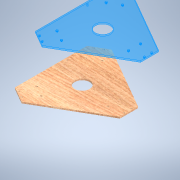
# Autodesk Inventor part: lep_felso
Saved by Autodesk Inventor 2022 (Build 260153000, 153)
## iProperties
Created: 2021-10-06
Part Number: lep_felso
Material: Wood (Birch)
Document SubType Name: Modeling
Designer: Varga Tamás
Density: 0.55 g/cm^3
Appearance: Birch - Natural Polished
Mass: 135.42 g
Surface Area: 1049.92 cm^2
Volume: 246.217 cm^3
Author: Varga Tamás
Autodesk Inventor part; units mm, degrees
ref_plane "YZ Plane" through (0, 0, 0) normal (1, 0, 0) x (0, 1, 0)
ref_plane "XZ Plane" through (0, 0, 0) normal (0, 1, 0) x (-1, 0, 0)
ref_plane "XY Plane" through (0, 0, 0) normal (0, 0, 1) x (1, 0, 0)
sketch "Sketch1" plane through (0, 0, 0) normal (0, 1, 0) x (-1, 0, 0)
  line L0 (-259.8076, 150) -> (-259.8076, 90)
  line L1 (-259.8076, 90) -> (-51.9615, -30)
  line L2 (-51.9615, -30) -> (0, 0)
  line L3 (0, 0) -> (0, 240)
  line L4 (0, 240) -> (-51.9615, 270)
  line L5 (-51.9615, 270) -> (-259.8076, 150)
  dimension "d0" = 120
  dimension "d1" = 120
  dimension "d2" = 120
  dimension "d4" = 120
  dimension "d5" = 120
  dimension "d6" = 60
  dimension "d7" = 120
  constraints: 13 end point, 2 equal length, 1 vertical
  measures "d0" angle of L4 L5
  measures "d1" angle of L3 L2
  measures "d2" angle of L1 L0
  measures "d4" angle of L1 L2
  measures "d5" angle of L3 L4
  measures "d6" distance of L0.start L0.end
  measures "d7" vertical distance of L4.end L0.start
extrude "Extrusion1" add sketch "Sketch1" along normal blind 5
sketch "Sketch2" plane through (0, 5, 0) normal (0, 1, 0) x (1, 0, 0)
  line L0 (254.8076, -108) -> (254.8076, -132)
  line L1 (259.8076, -150) -> (259.8076, -90) projected
  line L2 (259.8076, -90) -> (51.9615, 30) projected
  line L3 (51.9615, -270) -> (259.8076, -150) projected
  line L4 (209.8076, -108) -> (209.8076, -132)
  line L5 (209.8076, -108) -> (209.8076, -100)
  line L6 (209.8076, -144.7569) -> (209.8076, -140)
  point P0 (0, 0)
  dimension "d10" = 24
  dimension "d11" = 5
  dimension "d12" = 18
  dimension "d31" = 18.0885
  dimension "d32" = 18.0885
  dimension "d33" = 18
  dimension "d44" = 45
  dimension "d45" = 0
  dimension "d47" = 40.5885
  dimension "d51" = 8
  dimension "d52" = 8
  constraints: 8 end point, 6 coincident, 3 vertical, 2 parallel, 1 collinear
  measures "d10" distance of L0.start L0.end
  measures "d11" distance between parallel lines of L1 L0
  measures "d12" vertical distance of L1.end L0.start
  measures "d31" distance from line of L2 L0.start
  measures "d32" distance from line of L3 L0.end
  measures "d33" vertical distance of L1.start L0.end
  measures "d44" distance between parallel lines of L0 L4
  measures "d45" vertical distance of L0.start L4.start
  measures "d47" distance from line of L2 L4.start
  measures "d51" distance of L5.start L5.end
  measures "d52" distance of point (209.808, -132) L6.end
hole "Hole1" at (209.8076, 5, 100) at (209.8076, 5, 140) at (254.8076, 5, 108) at (254.8076, 5, 132) direction (0, -1, 0) diameter 2.8 end through all
sketch "Sketch3" plane through (0, 5, 0) normal (0, 1, 0) x (1, 0, 0)
  line L0 (18.088, 4.6696) -> (38.8735, 16.6701)
  line L1 (51.9615, 30) -> (0, 0) projected
  line L2 (0, 0) -> (0, -240) projected
  line L3 (259.8076, -90) -> (51.9615, 30) projected
  line L4 (47.516, -30.3017) -> (68.3015, -18.3011)
  line L5 (68.3015, -18.3011) -> (68.3015, -18.3011)
  line L6 (47.516, -30.3017) -> (33.66, -38.3014)
  dimension "d20" = 5
  dimension "d22" = 18.088
  dimension "d23" = 18.088
  dimension "d46" = 45
  dimension "d48" = 33.66
  dimension "d53" = 33.66
  dimension "d89" = 33.66
  constraints: 8 end point, 6 coincident, 3 parallel, 2 collinear
  measures "d20" distance from line of L1.end L0
  measures "d22" distance from line of L0.start L2
  measures "d23" distance from line of L3 L0.end
  measures "d46" distance between parallel lines of L4 L0
  measures "d48" distance from line of L3 L4.end
  measures "d53" distance from line of L3 L5.end
  measures "d89" distance from line of L2 point (33.66, -38.301)
hole "Hole2" at (68.3015, 5, 18.3011) at (33.66, 5, 38.3014) at (18.088, 5, -4.6696) at (38.8735, 5, -16.6701) direction (0, -1, 0) diameter 2.8 end through all
sketch "Sketch4" plane through (0, 5, 0) normal (0, 1, 0) x (1, 0, 0)
  line L0 (18.088, -244.6696) -> (38.8735, -256.6701)
  line L1 (0, -240) -> (51.9615, -270) projected
  line L2 (51.9615, -270) -> (259.8076, -150) projected
  line L3 (0, 0) -> (0, -240) projected
  line L4 (47.516, -209.6983) -> (68.3015, -221.6989)
  line L5 (68.3015, -221.6989) -> (68.3015, -221.6989)
  line L6 (47.516, -209.6983) -> (33.66, -201.6986)
  dimension "d34" = 5
  dimension "d35" = 18.088
  dimension "d36" = 18.088
  dimension "d49" = 45
  dimension "d50" = 33.66
  dimension "d56" = 33.66
  dimension "d90" = 33.66
  constraints: 8 end point, 6 coincident, 3 parallel, 2 collinear
  measures "d34" distance between parallel lines of L1 L0
  measures "d35" distance from line of L2 L0.end
  measures "d36" distance from line of L3 L0.start
  measures "d49" distance between parallel lines of L4 L0
  measures "d50" distance from line of L2 L4.end
  measures "d56" distance from line of L2 L5.end
  measures "d90" distance from line of L3 point (33.66, -201.699)
hole "Hole3" at (68.3015, 5, 221.6989) at (33.66, 5, 201.6986) at (18.088, 5, 244.6696) at (38.8735, 5, 256.6701) direction (0, -1, 0) diameter 2.8 end through all
sketch "Sketch5" plane through (0, 5, 0) normal (0, 1, 0) x (1, 0, 0)
  circle A0 centre (103.923, -120) radius 25
  line L0 (0, 0) -> (0, -240) projected
  line L1 (259.8076, -90) -> (51.9615, 30) projected
  line L2 (51.9615, 30) -> (0, 0) projected
  line L3 (25.9808, 15) -> (155.8846, -210)
  line L4 (51.9615, -270) -> (259.8076, -150) projected
  line L5 (51.9615, 30) -> (0, 0) projected
  line L6 (0, 0) -> (0, -240) projected
  line L7 (0, -120) -> (259.8076, -120)
  line L8 (259.8076, -150) -> (259.8076, -90) projected
  line L9 (0, -240) -> (51.9615, -270) projected
  line L10 (25.9808, -255) -> (155.8846, -30)
  dimension "d57" = 50
  dimension "d60" = 0
  dimension "d61" = 0
  constraints: 6 end point, 6 midpoint, 2 perpendicular, 1 centre point
  measures "d57" diameter of A0
  measures "d60" distance from line of A0.centre L7
  measures "d61" distance from line of L3 A0.centre
extrude "Extrusion2" cut sketch "Sketch5" against normal through all contours L7 L10 A0 | A0 L3 L7 | L10 L3 A0 | A0 L10 L3 | L7 A0 L3 | L10 A0 L7
sketch "Sketch6" plane through (0, 5, 0) normal (0, 1, 0) x (1, 0, 0)
  circle A0 centre (103.923, -120) radius 25 projected
  circle A1 centre (18.088, -244.6696) radius 1.4 projected
  circle A2 centre (68.3015, -221.6989) radius 1.4 projected
  circle A3 centre (33.66, -201.6986) radius 1.4 projected
  circle A4 centre (38.8735, -256.6701) radius 1.4 projected
  circle A5 centre (18.088, 4.6696) radius 1.4 projected
  circle A6 centre (68.3015, -18.3011) radius 1.4 projected
  circle A7 centre (33.66, -38.3014) radius 1.4 projected
  circle A8 centre (38.8735, 16.6701) radius 1.4 projected
  circle A9 centre (254.8076, -108) radius 1.4 projected
  circle A10 centre (209.8076, -100) radius 1.4 projected
  circle A11 centre (209.8076, -140) radius 1.4 projected
  circle A12 centre (254.8076, -132) radius 1.4 projected
  line L0 (259.8076, -90) -> (51.9615, 30) projected
  line L1 (51.9615, 30) -> (0, 0) projected
  line L2 (0, 0) -> (0, -240) projected
  line L3 (0, -240) -> (51.9615, -270) projected
  line L4 (51.9615, -270) -> (259.8076, -150) projected
  line L5 (259.8076, -150) -> (259.8076, -90) projected
  line L6 (36.3641, -199.5334) -> (36.8871, -202.9578)
  line L7 (36.8871, -202.9578) -> (34.183, -205.123)
  line L8 (34.183, -205.123) -> (30.9559, -203.8638)
  line L9 (30.9559, -203.8638) -> (30.4329, -200.4394)
  line L10 (30.4329, -200.4394) -> (33.137, -198.2742)
  line L11 (33.137, -198.2742) -> (36.3641, -199.5334)
  circle A13 centre (68.3015, -221.6989) radius 1.4 projected
  line L12 (67.8588, -218.2632) -> (71.0556, -219.5976)
  line L13 (71.0556, -219.5976) -> (71.4983, -223.0333)
  line L14 (71.4983, -223.0333) -> (68.7442, -225.1346)
  line L15 (68.7442, -225.1346) -> (65.5475, -223.8001)
  line L16 (65.5475, -223.8001) -> (65.1048, -220.3644)
  line L17 (65.1048, -220.3644) -> (67.8588, -218.2632)
  circle A14 centre (209.8076, -140) radius 1.4 projected
  line L18 (212.8076, -138.2679) -> (212.8076, -141.7321)
  line L19 (212.8076, -141.7321) -> (209.8076, -143.4641)
  line L20 (209.8076, -143.4641) -> (206.8076, -141.7321)
  line L21 (206.8076, -141.7321) -> (206.8076, -138.2679)
  line L22 (206.8076, -138.2679) -> (209.8076, -136.5359)
  line L23 (209.8076, -136.5359) -> (212.8076, -138.2679)
  line L24 (206.8076, -98.2679) -> (209.8076, -96.5359)
  line L25 (209.8076, -96.5359) -> (212.8076, -98.2679)
  line L26 (212.8076, -98.2679) -> (212.8076, -101.7321)
  line L27 (212.8076, -101.7321) -> (209.8076, -103.4641)
  line L28 (209.8076, -103.4641) -> (206.8076, -101.7321)
  line L29 (206.8076, -101.7321) -> (206.8076, -98.2679)
  circle A15 centre (68.3015, -18.3011) radius 1.4 projected
  line L30 (69.9304, -15.2439) -> (71.7636, -18.1831)
  line L31 (71.7636, -18.1831) -> (70.1348, -21.2404)
  line L32 (70.1348, -21.2404) -> (66.6727, -21.3584)
  line L33 (66.6727, -21.3584) -> (64.8394, -18.4191)
  line L34 (64.8394, -18.4191) -> (66.4683, -15.3619)
  line L35 (66.4683, -15.3619) -> (69.9304, -15.2439)
  circle A16 centre (33.66, -38.3014) radius 1.4 projected
  line L36 (33.66, -34.8373) -> (36.66, -36.5694)
  line L37 (36.66, -36.5694) -> (36.66, -40.0335)
  line L38 (36.66, -40.0335) -> (33.66, -41.7655)
  line L39 (33.66, -41.7655) -> (30.66, -40.0335)
  line L40 (30.66, -40.0335) -> (30.66, -36.5694)
  line L41 (30.66, -36.5694) -> (33.66, -34.8373)
  line L42 (0, 0) -> (0, -240) projected
  line L43 (51.9615, -270) -> (259.8076, -150) projected
  line L44 (259.8076, -90) -> (51.9615, 30) projected
  circle A17 centre (18.088, -244.6696) radius 3
  circle A18 centre (38.8735, -256.6701) radius 3
  circle A19 centre (18.088, 4.6696) radius 3
  circle A20 centre (38.8735, 16.6701) radius 3
  circle A21 centre (254.8076, -108) radius 3
  circle A22 centre (254.8076, -132) radius 3
  dimension "d66" = 6
  dimension "d67" = 6
  dimension "d68" = 6
  dimension "d71" = 6
  dimension "d72" = 6
  dimension "d73" = 6
  dimension "d78" = 6
  dimension "d79" = 6
  dimension "d80" = 6
  dimension "d81" = 6
  dimension "d82" = 6
  dimension "d83" = 6
  constraints: 72 end point, 13 coincident, 6 centre point, 3 parallel, 1 point on line, 78 other
  measures "d66" distance between parallel lines of L41 L38
  measures "d67" distance between parallel lines of L35 L32
  measures "d68" distance between parallel lines of L24 L27
  measures "d71" distance between parallel lines of L21 L18
  measures "d72" distance between parallel lines of L15 L12
  measures "d73" distance between parallel lines of L9 L6
  measures "d78" diameter of A17
  measures "d79" diameter of A18
  measures "d80" diameter of A19
  measures "d81" diameter of A20
  measures "d82" diameter of A21
  measures "d83" diameter of A22
extrude "Extrusion3" cut sketch "Sketch6" against normal blind 2.5 contours A1 | A4 | A5 | A6 | A8 | A9 | A10 | A11 | A12 | L6 L7 L8 L9 L10 L11 | L12 L13 L14 L15 L16 L17 | L18 L19 L20 L21 L22 L23 | L24 L25 L26 L27 L28 L29 | L30 L31 L32 L33 L34 L35 | L36 L37 L38 L39 L40 L41 | A17 | A18 | A19 | A20 | A21 | A22
sketch "Sketch7" plane through (0, 5, 0) normal (0, 1, 0) x (1, 0, 0)
  circle A0 centre (7.9, -75) radius 2.5
  line L0 (0, 0) -> (0, -240) projected
  dimension "d84" = 75
  dimension "d85" = 5
  dimension "d88" = 7.9
  constraints: 1 centre point
  measures "d84" vertical distance of L0.start A0.centre
  measures "d85" diameter of A0
  measures "d88" distance from line of L0 A0.centre
extrude "Extrusion4" cut sketch "Sketch7" against normal through all
body "Solid1"
